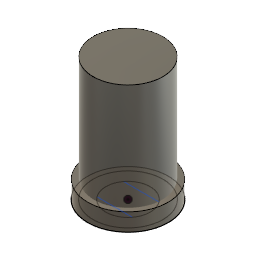
arm_stepper_connector v1 (Autodesk Fusion 360 design; units mm, degrees)
Autodesk Fusion 360 part; units mm, degrees
sketch "Sketch1" plane through (0, 0, 0) normal (0, 1, 0) x (1, 0, 0)
  circle A0 centre (0, 0) radius 3.95
  circle A1 centre (0, 0) radius 2.5
  line L0 (0, 1.5) -> (2, 1.5)
  line L1 (0, 1.5) -> (-2, 1.5)
  line L2 (0, -1.5) -> (-2, -1.5)
  line L3 (0, -1.5) -> (2, -1.5)
  circle A2 centre (0, 0) radius 4.55
  dimension "d1" = 7.9
  dimension "d2" = 5
  dimension "d3" = 9.1
  measures "d1" diameter of A0
  measures "d2" diameter of A1
  measures "d3" diameter of A2
extrude "Extrude2" add sketch "Sketch1" along normal blind 14 contours A0 | A1 L0 L1 L2 L3 | A1 L0 L1 | A1 L2 L3 makes body 1
extrude "Extrude1" add sketch "Sketch1" along normal blind 2 separate body contours A0 | A1 L0 L1 L2 L3 | A1 L0 L1 | A1 L2 L3 | A2 makes body 2
extrude "Extrude3" cut sketch "Sketch1" along normal blind 1.55 contours A0 bodies 1 2
extrude "Extrude4" cut sketch "Sketch1" along normal blind 10 contours A1 L0 L1 L2 L3 bodies 1 2
extrude "Extrude5" cut sketch "Sketch1" along normal blind 4.05 contours A1 L0 L1 | A1 L2 L3 bodies 1 2
